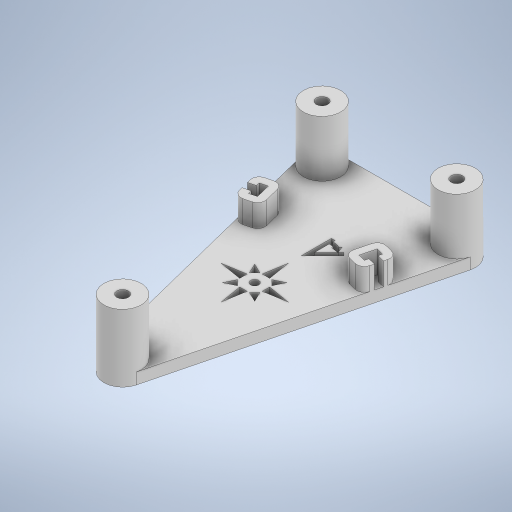
# Autodesk Inventor part: BaseLiDARv2
Saved by Autodesk Inventor 2024.2 (Build 282272000, 272)
## iProperties
Created: 2024-07-17
Part Number: BaseLiDARv2
Material: Generic
Document SubType Name: Modeling
Designer: jrcer
Density: 1 g/cm^3
Appearance: Default
Author: jrcer
Autodesk Inventor part; units mm, degrees
ref_plane "YZ Plane" through (0, 0, 0) normal (1, 0, 0) x (0, 1, 0)
ref_plane "XZ Plane" through (0, 0, 0) normal (0, 1, 0) x (-1, 0, 0)
ref_plane "XY Plane" through (0, 0, 0) normal (0, 0, 1) x (1, 0, 0)
sketch "Sketch1" plane through (0, 0, 0) normal (0, 1, 0) x (-1, 0, 0)
  circle A0 centre (0, 35.3) radius 1.55
  circle A1 centre (18, -36) radius 1.55
  circle A2 centre (-18, -36) radius 1.55
  circle A3 centre (0, 35.3) radius 5
  circle A4 centre (18, -36) radius 5
  circle A5 centre (-18, -36) radius 5
  point P0 (0, 0)
  dimension "d0" = 35.3
  dimension "d1" = 36
  dimension "d2" = 3.1
  dimension "d3" = 10
  dimension "d4" = 36
  dimension "d5" = 18
  constraints: 6 centre point, 4 equal radius, 3 coincident, 1 horizontal alignment, 1 vertical alignment
  measures "d0" distance of A0.centre point (0, 0)
  measures "d1" vertical distance of A2.centre point (0, 0)
  measures "d2" diameter of A0
  measures "d3" diameter of A3
  measures "d4" distance of A2.centre A1.centre
  measures "d5" horizontal distance of point (0, 0) A2.centre
extrude "Extrusion1" add sketch "Sketch1" along normal blind 15
sketch "Sketch2" plane through (0, 0, 35.3) normal (0, -1, 0) x (1, 0, 0)
  circle A0 centre (0, 0) radius 5 projected
  circle A1 centre (0, 0) radius 1.55 projected
  circle A2 centre (-18, -71.3) radius 1.55 projected
  circle A3 centre (-18, -71.3) radius 5 projected
  circle A4 centre (18, -71.3) radius 1.55 projected
  circle A5 centre (18, -71.3) radius 5 projected
  line L0 (-22.8479, -70.0761) -> (-4.8479, 1.2239)
  line L1 (22.8479, -70.0761) -> (4.8479, 1.2239)
  line L2 (-18, -76.3) -> (18, -76.3)
  circle A6 centre (0, -35.3) radius 1.1
  dimension "d8" = 2.2
  constraints: 6 end point, 6 point on circle, 5 tangent, 1 centre point, 1 coincident, 1 horizontal
  measures "d8" diameter of A6
extrude "Extrusion2" add sketch "Sketch2" along normal blind 3
sketch "Sketch3" plane through (0, 0, 35.3) normal (0, 1, 0) x (1, 0, 0)
  circle A0 centre (0, 35.3) radius 1.1 construction
  line L0 (0, 44.3) -> (1, 38.3)
  line L1 (1, 38.3) -> (-1, 38.3)
  line L2 (-3, 36.3) -> (-9, 35.3)
  line L3 (-1, 38.3) -> (0, 44.3)
  line L4 (-9, 35.3) -> (-3, 34.3)
  line L5 (-3, 34.3) -> (-3, 36.3)
  line L6 (1.1, 35.3) -> (-1.1, 35.3) construction
  line L7 (0, 36.4) -> (0, 34.2) construction
  line L8 (3, 36.3) -> (9, 35.3)
  line L9 (9, 35.3) -> (3, 34.3)
  line L10 (3, 34.3) -> (3, 36.3)
  line L11 (0, 26.3) -> (1, 32.3)
  line L12 (1, 32.3) -> (-1, 32.3)
  line L13 (-1, 32.3) -> (0, 26.3)
  line L14 (-0.7778, 36.0778) -> (0.7778, 34.5222) construction
  line L15 (0.7778, 36.0778) -> (-0.7778, 34.5222) construction
  line L16 (-4.2929, 39.5929) -> (-3, 36.8858)
  line L17 (-3, 36.8858) -> (-1.5858, 38.3)
  line L18 (-1.5858, 38.3) -> (-4.2929, 39.5929)
  line L19 (-0.7778, 36.0778) -> (-4.2929, 39.5929) construction
  line L20 (4.2929, 39.5929) -> (3, 36.8858)
  line L21 (3, 36.8858) -> (1.5858, 38.3)
  line L22 (1.5858, 38.3) -> (4.2929, 39.5929)
  line L23 (-4.2929, 31.0071) -> (-3, 33.7142)
  line L24 (-3, 33.7142) -> (-1.5858, 32.3)
  line L25 (-1.5858, 32.3) -> (-4.2929, 31.0071)
  line L26 (4.2929, 31.0071) -> (3, 33.7142)
  line L27 (1.5858, 32.3) -> (4.2929, 31.0071)
  line L28 (3, 33.7142) -> (1.5858, 32.3)
  point P0 (0, 38.3)
  point P1 (0, 32.3)
  point P2 (0, 35.3)
  point P3 (-2.2929, 37.5929)
  dimension "d11" = 3
  dimension "d12" = 6
  dimension "d13" = 2
  dimension "d14" = 3
  dimension "d15" = 45
  dimension "d16" = 45
  dimension "d17" = 3
  constraints: 58 end point, 16 symmetric about line, 7 midpoint, 5 equal length, 3 horizontal alignment, 3 vertical alignment, 2 horizontal, 1 collinear, 1 perpendicular, 1 point on line, 1 vertical, 9 other
  measures "d11" distance from line of point (0, 35.3) L1
  measures "d12" distance of point (0, 38.3) L0.start
  measures "d13" distance of L0.end L1.end
  measures "d14" distance between parallel lines of L7 L5
  measures "d15" angle of L6 L14
  measures "d16" angle of L6 L15
  measures "d17" distance of L17.end L16.start
extrude "Extrusion3" cut sketch "Sketch3" against normal blind 3
sketch "Sketch4" plane through (0, 0, 35.3) normal (0, 1, 0) x (1, 0, 0)
  line L0 (0, 55.8) -> (0, 47.8)
  line L1 (0, 47.8) -> (5.6569, 53.4569)
  line L2 (4.9497, 54.164) -> (1, 50.2142)
  line L3 (1, 50.2142) -> (1, 55.8)
  line L4 (0, 55.8) -> (1, 55.8)
  line L5 (4.9497, 54.164) -> (5.6569, 53.4569)
  arc A0 (3.8284, 53.0426) -> (1, 54.2142) centre (1, 50.2142) ccw
  arc A1 (4.5355, 53.7497) -> (1, 55.2142) centre (1, 50.2142) ccw
  line L6 (4.182, 53.3962) -> (2.1997, 53.6617)
  line L7 (2.1997, 53.6617) -> (3.4208, 55.2457)
  line L8 (3.4208, 55.2457) -> (4.182, 53.3962)
  arc A2 (4.182, 53.3962) -> (1, 54.7142) centre (1, 50.2142) ccw construction
  point P0 (0, 35.3)
  point P1 (3.2675, 54.1012)
  point P2 (2.4237, 53.9523)
  point P3 (3.0557, 54.7721)
  point P4 (3.2507, 53.5209)
  point P5 (3.7816, 54.3691)
  dimension "d21" = 45
  dimension "d22" = 8
  dimension "d23" = 12.5
  dimension "d24" = 1
  dimension "d25" = 4
  dimension "d26" = 5
  dimension "d27" = 4.5
  dimension "d28" = 2
  constraints: 18 end point, 7 point on circle, 6 point on line, 3 centre point, 3 coincident, 1 equal length, 1 horizontal, 1 perpendicular, 1 vertical, 1 vertical alignment, 6 other
  measures "d21" angle of L0 L1
  measures "d22" distance of L0.start L0.end
  measures "d23" distance of L0.end point (0, 35.3)
  measures "d24" distance between parallel lines of L1 L2
  measures "d25" radius of A0
  measures "d26" radius of A1
  measures "d27" radius of A2
  measures "d28" distance of L6.start L6.end
extrude "Extrusion4" cut sketch "Sketch4" against normal blind 1.5 contours L4 L3 L2 L5 L1 L0 | A1 L7 A0 L3 | L7 L8 A1 | A1 L8 L6 A0 L7 | A0 L6 L7
sketch "Sketch5" plane through (0, 0, 35.3) normal (0, 1, 0) x (1, 0, 0)
  circle A0 centre (18, 71.3) radius 1.55 construction
  line L0 (22.8479, 70.0761) -> (4.8479, -1.2239) construction
  line L1 (13.084, 55.9126) -> (18.9015, 54.444)
  line L2 (18.9015, 54.444) -> (16.9433, 46.6874)
  line L3 (16.9433, 46.6874) -> (11.1258, 48.156)
  line L4 (11.1258, 48.156) -> (13.084, 55.9126)
  line L5 (11.1258, 48.156) -> (18.9015, 54.444) construction
  line L6 (16.9433, 46.6874) -> (13.084, 55.9126) construction
  line L7 (13.5545, 49.6056) -> (15.4937, 49.1161)
  line L8 (15.4937, 49.1161) -> (16.4728, 52.9944)
  line L9 (16.4728, 52.9944) -> (14.5336, 53.4839)
  line L10 (14.5336, 53.4839) -> (13.5545, 49.6056)
  line L11 (17.6776, 49.5961) -> (15.7385, 50.0856)
  line L12 (18.1672, 51.5353) -> (16.228, 52.0248)
  line L13 (0, 47.8) -> (0, 55.8) construction
  line L14 (-13.084, 55.9126) -> (-18.9015, 54.444)
  line L15 (-18.9015, 54.444) -> (-16.9433, 46.6874)
  line L16 (-16.9433, 46.6874) -> (-11.1258, 48.156)
  line L17 (-11.1258, 48.156) -> (-13.084, 55.9126)
  line L18 (-11.1258, 48.156) -> (-18.9015, 54.444) construction
  line L19 (-16.9433, 46.6874) -> (-13.084, 55.9126) construction
  line L20 (-13.5545, 49.6056) -> (-15.4937, 49.1161)
  line L21 (-15.4937, 49.1161) -> (-16.4728, 52.9944)
  line L22 (-16.4728, 52.9944) -> (-14.5336, 53.4839)
  line L23 (-14.5336, 53.4839) -> (-13.5545, 49.6056)
  line L24 (-17.6776, 49.5961) -> (-15.7385, 50.0856)
  line L25 (-18.1672, 51.5353) -> (-16.228, 52.0248)
  point P0 (0, 35.3)
  point P1 (15.0137, 51.3)
  point P2 (15.0137, 51.3)
  point P3 (-15.0137, 51.3)
  point P4 (-15.0137, 51.3)
  dimension "d31" = 8
  dimension "d32" = 20
  dimension "d33" = 6
  dimension "d34" = 2
  dimension "d35" = 3
  dimension "d36" = 3
  constraints: 48 end point, 14 symmetric about line, 9 point on line, 4 parallel, 4 perpendicular, 2 midpoint, 1 collinear, 3 other
  measures "d31" distance of L3.end L1.start
  measures "d32" vertical distance of A0.centre point (15.014, 51.3)
  measures "d33" distance of L1.start L1.end
  measures "d34" distance between parallel lines of L3 L7
  measures "d35" distance between parallel lines of L3 L11
  measures "d36" distance between parallel lines of L1 L12
extrude "Extrusion5" add sketch "Sketch5" along normal blind 6 contours L1 L2 L12 L8 L9 L10 L7 L11 L3 L4 | L17 L16 L15 L24 L21 L20 L23 L22 L25 L14
fillet "Fillet1" radius 2 8 edges at (-11.1258, 3, -12.856) (-16.9433, 3, -11.3874) (-13.084, 3, -20.6126) (16.9433, 3, -11.3874) (11.1258, 3, -12.856) (18.9015, 3, -19.144) (-18.9015, 3, -19.144) (13.084, 3, -20.6126)
equation "\"d5\" = 0.5 * d4"
equation "\"d14\" = d11"
equation "\"d36\" = d35"
body "Solid1"
